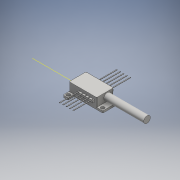
# Autodesk Inventor part: gainchip
Saved by Autodesk Inventor 2016 (Build 200138000, 138)
## iProperties
Created: 2015-09-04
Part Number: gainchip
Material: Generic
Document SubType Name: Modeling
Designer: HE BEC
Density: 1 g/cm^3
Appearance: Default
Author: HE BEC
Autodesk Inventor part; units mm, degrees
ref_plane "YZ Plane" through (0, 0, 0) normal (1, 0, 0) x (0, 1, 0)
ref_plane "XZ Plane" through (0, 0, 0) normal (0, 1, 0) x (-1, 0, 0)
sketch "Sketch1" plane through (0, 0, 0) normal (0, 0, 1) x (1, 0, 0)
  line L0 (-10.4, -6.35) -> (10.4, -6.35)
  line L1 (10.4, -6.35) -> (10.4, 6.35)
  line L2 (10.4, 6.35) -> (-10.4, 6.35)
  line L3 (-10.4, 6.35) -> (-10.4, -6.35)
  line L4 (-10.4, -6.35) -> (10.4, 6.35) construction
  line L5 (10.4, -6.35) -> (-10.4, 6.35) construction
  point P0 (0, 0)
  dimension "d0" = 12.7
  dimension "d1" = 20.8
  constraints: 12 end point, 2 midpoint, 2 parallel, 1 horizontal, 1 perpendicular
  measures "d0" distance of L0.end L1.end
  measures "d1" distance of L1.end L2.end
extrude "Extrusion1" add sketch "Sketch1" along normal blind 6.4
sketch "Sketch4" plane through (0, 0, 0) normal (0, 0, -1) x (-1, 0, 0)
  line L0 (10.4, -10.95) -> (6.6, -10.95)
  line L1 (-15, -6.35) -> (-15, 0)
  line L2 (-15, 0) -> (10.4, 0)
  line L3 (10.4, 0) -> (10.4, -10.95)
  line L4 (10.4, 6.35) -> (10.4, -6.35) projected
  line L5 (-15, -6.35) -> (6.6, -6.35)
  line L6 (6.6, -6.35) -> (6.6, -10.95)
  line L7 (10.4, -6.35) -> (-10.4, -6.35) projected
  point P0 (0, 0)
  dimension "d18" = 10.95
  dimension "d20" = 25.4
  dimension "d21" = 3.8
  constraints: 12 end point, 4 parallel, 1 horizontal, 1 midpoint, 1 perpendicular, 1 point on line
  measures "d18" distance of L2.end L0.start
  measures "d20" distance between parallel lines of L1 L3
  measures "d21" distance of L0.start L0.end
extrude "Extrusion4" add sketch "Sketch4" along normal blind 1.5
sketch "Sketch5" plane through (0, 0, -1.5) normal (0, 0, -1) x (-1, 0, 0)
  circle A0 centre (8.5, -8.95) radius 1.35
  circle A1 centre (-13, -4.45) radius 1.35
  line L0 (6.6, -10.95) -> (10.4, -10.95) projected
  line L1 (10.4, 0) -> (-15, 0) projected
  line L2 (10.4, -10.95) -> (10.4, 0) projected
  line L3 (-15, 0) -> (-15, -6.35) projected
  line L4 (-15, -6.35) -> (6.6, -6.35) projected
  point P0 (0, 0)
  dimension "d24" = 2.7
  dimension "d26" = 8.95
  dimension "d28" = 1.9
  dimension "d29" = 2
  dimension "d31" = 4.45
  constraints: 2 centre point, 1 equal radius
  measures "d24" diameter of A0
  measures "d26" distance from line of L1 A0.centre
  measures "d28" distance from line of L2 A0.centre
  measures "d29" distance from line of L3 A1.centre
  measures "d31" distance from line of L1 A1.centre
extrude "Extrusion5" cut sketch "Sketch5" against normal through all
chamfer "Chamfer2" distance 0.5 angle 45 3 edges at (-10.4, -10.95, -0.75) (-6.6, -10.95, -0.75) (15, -6.35, -0.75)
mirror "Mirror3" about plane through (0, 0, 0) normal (0, 1, 0) of "Extrusion4", "Extrusion5", "Chamfer2"
fillet "Fillet1" radius 0.5 4 edges at (10.4, -6.35, 3.2) (-10.4, -6.35, 3.2) (-10.4, 6.35, 3.2) (10.4, 6.35, 3.2)
ref_plane "Work Plane2" through (0, 0, 2.665) normal (0, 0, -1) x (-1, 0, 0)
sketch "Sketch6" plane through (0, 0, 2.665) normal (0, 0, -1) x (-1, 0, 0)
  line L0 (-9.9, 6.35) -> (9.9, 6.35) projected
  line L1 (-8.8, 6.35) -> (3.2, 6.35)
  line L2 (3.2, 6.35) -> (3.2, 7.65)
  line L3 (3.2, 7.65) -> (-8.8, 7.65)
  line L4 (-8.8, 7.65) -> (-8.8, 6.35)
  line L5 (-10.4, -5.85) -> (-10.4, 5.85) projected
  point P0 (0, 0)
  dimension "d39" = 1.3
  dimension "d40" = 12
  dimension "d41" = 1.6
  constraints: 8 end point, 2 parallel, 1 horizontal, 1 perpendicular, 1 point on line
  measures "d39" distance of L3.end L1.start
  measures "d40" distance of L2.end L3.end
  measures "d41" distance between parallel lines of L5 L4
extrude "Extrusion6" add sketch "Sketch6" against normal blind 1.5
sketch "Sketch7" plane through (0, 0, 4.165) normal (0, 0, 1) x (1, 0, 0)
  line L0 (8.8, 6.35) -> (-3.2, 6.35) projected
  line L1 (8.12, 6.35) -> (7.62, 6.35)
  line L2 (7.62, 6.35) -> (7.62, 21.65)
  line L3 (7.62, 21.65) -> (8.12, 21.65)
  line L4 (8.12, 21.65) -> (8.12, 6.35)
  line L5 (-15.48, 0) -> (20.08, 0) projected
  line L6 (7.87, 6.35) -> (7.87, 21.65) construction
  line L7 (10.4, -5.85) -> (10.4, 5.85) projected
  point P0 (0, 0)
  dimension "d46" = 21.65
  dimension "d47" = 2.53
  dimension "d48" = 0.5
  constraints: 10 end point, 3 parallel, 2 midpoint, 1 horizontal, 1 perpendicular, 1 point on line
  measures "d46" distance between parallel lines of L3 L5
  measures "d47" distance between parallel lines of L7 L6
  measures "d48" distance of L2.end L3.end
extrude "Extrusion7" add sketch "Sketch7" along normal blind 0.2
pattern_linear "Rectangular Pattern1" count 5 spacing 2.54 along (-1, 0, 0) of "Extrusion7"
mirror "Mirror4" about plane through (0, 0, 0) normal (0, 1, 0) of "Extrusion6", "Extrusion7", "Rectangular Pattern1"
sketch "Sketch8" plane through (-10.4, -10.45, -1.5) normal (-1, 0, 0) x (0, 0, 1)
  line L0 (0, 0) -> (0, 20.9) projected
  line L1 (1.5, 4.1) -> (7.9, 4.1) projected
  point P0 (1.5, 10.45)
  point P1 (4.8, 8.6)
  dimension "d54" = 4.8
  dimension "d55" = 4.5
  measures "d54" distance from line of L0 point (4.8, 8.6)
  measures "d55" distance from line of L1 point (4.8, 8.6)
sketch "Sketch9" plane through (10.4, -5.85, 6.4) normal (1, 0, 0) x (0, 0, -1)
  line L0 (7.9, 0) -> (7.9, 11.7) projected
  line L1 (6.4, 12.2) -> (0, 12.2) projected
  circle A0 centre (3.2, 7.35) radius 2.5
  point P0 (6.4, 5.85)
  dimension "d56" = 4.7
  dimension "d57" = 4.85
  dimension "d58" = 5
  constraints: 1 centre point, 1 coincident
  measures "d56" distance from line of L0 point (3.2, 7.35)
  measures "d57" distance from line of L1 point (3.2, 7.35)
  measures "d58" diameter of A0
extrude "fibre_connect" add sketch "Sketch9" along normal blind 30.15
ref_plane "Work Plane1" through (0, 0, 0) normal (0, 1, 0) x (-1, 0, 0)
ref_plane "Work Plane3" through (0, 0, 0) normal (0, 1, 0) x (-1, 0, 0)
body "Solid1"
